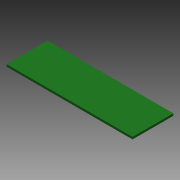
# Autodesk Inventor part: NoiseBoard
Saved by Autodesk Inventor 2014 (Build 180170000, 170)
## iProperties
Created: 2015-11-05
Part Number: NoiseBoard
Material: Generic
Document SubType Name: Modeling
Designer: Owner
Density: 1 g/cm^3
Appearance: Smooth - Dark Forest Green
Author: Owner
Autodesk Inventor part; units mm, degrees
ref_plane "YZ Plane" through (0, 0, 0) normal (1, 0, 0) x (0, 1, 0)
ref_plane "XZ Plane" through (0, 0, 0) normal (0, 1, 0) x (-1, 0, 0)
ref_plane "XY Plane" through (0, 0, 0) normal (0, 0, 1) x (1, 0, 0)
sketch "Sketch1" plane through (0, 0, 0) normal (0, 1, 0) x (-1, 0, 0)
  line L0 (-9.7887, 9.8211) -> (84.1913, 9.8211)
  line L1 (84.1913, 9.8211) -> (84.1913, -20.6589)
  line L2 (84.1913, -20.6589) -> (-9.7887, -20.6589)
  line L3 (-9.7887, -20.6589) -> (-9.7887, 9.8211)
  line L4 (-9.7887, -13.5469) -> (3.9273, -13.5469)
  line L5 (3.9273, -13.5469) -> (7.7373, -17.3569)
  line L6 (7.7373, -17.3569) -> (28.8193, -17.3569)
  line L7 (28.8193, -17.3569) -> (32.1213, -20.6589)
  point P0 (0, 0)
  dimension "d0" = 93.98
  dimension "d1" = 30.48
  dimension "d4" = 45
  dimension "d5" = 21.082
  dimension "d6" = 13.716
  dimension "d7" = 45
  dimension "d8" = 23.368
  dimension "d9" = 27.178
  constraints: 16 end point, 3 parallel, 2 perpendicular, 2 point on line, 1 horizontal
  measures "d0" distance of L0.start L0.end
  measures "d1" distance of L2.end L0.start
  measures "d4" angle of L2 L7
  measures "d5" distance of L6.end L5.end
  measures "d6" distance of L4.start L4.end
  measures "d7" angle of L6 L5
  measures "d8" distance between parallel lines of L0 L4
  measures "d9" distance between parallel lines of L0 L6
extrude "Extrusion1" add sketch "Sketch1" along normal blind 1.6 contours L0 L1 L2 L7 L6 L5 L4 L3
body "Solid1"
